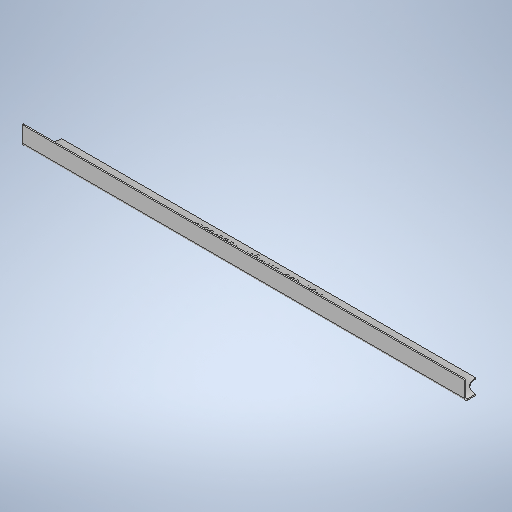
# Autodesk Inventor part: MSC 068 stringer lowerback
Saved by Autodesk Inventor 2025 (Build 290162010, 162A)
## iProperties
Created: 2024-04-28
Part Number: MSC 068 stringer lowerback
Material: Stainless Steel
Document SubType Name: Sheet Metal
Designer: admin
Stock Number: МОО 068 стрингер поясница
Density: 8 g/cm^3
Flat Pattern Width: 70 cm
Flat Pattern Length: 6.6202 cm
Flat Pattern Area: 463.414 cm^2
Sheet Metal Rule: AISI304 2mm Die16
Sheet Metal Width: 700,000 mm
Sheet Metal Length: 66,202 mm
Sheet Metal Area: 46341,393 mm^2
Appearance: Default
Author: admin
Autodesk Inventor part; units mm, degrees
ref_plane "YZ Plane" through (0, 0, 0) normal (1, 0, 0) x (0, 1, 0)
ref_plane "XZ Plane" through (0, 0, 0) normal (0, 1, 0) x (-1, 0, 0)
ref_plane "XY Plane" through (0, 0, 0) normal (0, 0, 1) x (1, 0, 0)
sketch "Sketch1" plane through (0, 0, 0) normal (0, 0, 1) x (1, 0, 0)
  line L0 (-700, 40) -> (0, 40)
  line L1 (0, 40) -> (0, 0)
  line L2 (0, 0) -> (-700, 0)
  line L3 (-700, 0) -> (-700, 40)
  point P0 (-350, 0)
  dimension "d1" = 40
  dimension "d45" = 700
  measures "d1" distance of L0.end L1.end
  measures "d45" distance of L1.end L2.end
extrude "Plate1" add sketch "Sketch1" along normal blind 2
sketch "Sketch2" plane through (0, 2, 0) normal (0, -1, 0) x (1, 0, 0)
  line L0 (-700, 0) -> (0, 0)
  line L1 (0, 0) -> (0, 30)
  line L2 (0, 30) -> (-700, 30)
  line L3 (-700, 30) -> (-700, 0)
  constraints: 6 end point, 1 horizontal, 1 perpendicular, 1 vertical
edge flange "Flange1" height 30 angle 90 thickness 2 bend radius 2.75 thickness toward (0, -1, 0) relief round relief width 2 relief depth 1 edges at (-350, 0, 2) wall of the first edge with corners at (-700, 2, 0) (0, 2, 0) (0, 2, 30) (-700, 2, 30)
bend "Bend1"
corner "Corner1"
sketch "Sketch6" plane through (0, 0, 0) normal (0, 0, -1) x (-1, 0, 0)
  line L0 (0, 40) -> (0, 4.75) projected
  circle A0 centre (0, 40) radius 22.5
  line L1 (0, 40) -> (700, 40) projected
  line L2 (-499, 30) -> (-499, 67.6691) projected
  point P0 (0, 0)
  point P1 (22.5, 40)
  point P2 (0, 17.5)
  dimension "d24" = 45
  constraints: 1 centre point, 1 other
  measures "d24" diameter of A0
extrude "Extrusion2" cut sketch "Sketch6" along normal mid plane 30 contours L1 A0 L0 picked at (14.812, 38.3311)
sketch "Sketch9" plane through (0, 0, 2) normal (0, 0, 1) x (1, 0, 0)
  line L0 (-256.9226, 35) -> (-256.9226, 23) construction
  line L1 (-256.9226, 23) -> (-456.9226, 23) construction
  line L2 (-456.9226, 23) -> (-456.9226, 35) construction
  line L3 (-456.9226, 35) -> (-256.9226, 35) construction
  line L4 (-700, 40) -> (0, 40) projected
  point P0 (0, 0)
  dimension "d40" = 200
  dimension "d41" = 12
  dimension "d43" = 5
  constraints: 2 other
  measures "d40" distance of L0.end L1.end
  measures "d41" distance of L1.end L2.end
  measures "d43" distance between parallel lines of L4 L3
mark "Mark2"
sketch "Sketch10" plane through (-700, 40, 2) normal (0, 0, 1) x (1, 0, 0)
  circle A0 centre (0, 0) radius 22.5
  line L0 (246.5218, -6.4882) -> (246.5218, -9.8215) projected
  line L1 (246.5218, -9.8215) -> (246.5218, -16.4882) projected
  line L2 (246.5218, -9.8215) -> (242.0774, -13.1549) projected
  line L3 (269.8552, -13.1549) -> (269.8552, -6.4882) projected
  line L4 (269.8552, -16.4882) -> (269.8552, -13.1549) projected
  line L5 (267.0774, -13.1549) -> (269.8552, -13.1549) projected
  arc A1 (265.4107, -11.4882) -> (267.0774, -13.1549) centre (267.0774, -11.4882) ccw projected
  line L6 (265.4107, -8.1549) -> (265.4107, -11.4882) projected
  arc A2 (267.0774, -6.4882) -> (265.4107, -8.1549) centre (267.0774, -8.1549) ccw projected
  line L7 (269.8552, -6.4882) -> (267.0774, -6.4882) projected
  line L8 (305.4107, -6.4882) -> (305.9663, -6.4882) projected
  arc A3 (307.6329, -8.1549) -> (305.9663, -6.4882) centre (305.9663, -8.1549) ccw projected
  line L9 (307.6329, -8.1549) -> (307.6329, -16.4882) projected
  circle A4 centre (351.244, -16.2104) radius 0.2778 projected
  line L10 (351.244, -6.4882) -> (351.244, -13.1549) projected
  line L11 (363.744, -6.4882) -> (363.744, -13.1549) projected
  line L12 (364.8552, -13.1549) -> (363.744, -13.1549) projected
  line L13 (363.744, -13.1549) -> (363.744, -16.4882) projected
  line L14 (363.744, -13.1549) -> (361.5218, -13.1549) projected
  line L15 (419.2996, -6.4882) -> (421.5218, -6.4882) projected
  arc A5 (423.744, -8.7104) -> (421.5218, -6.4882) centre (421.5218, -8.7104) ccw projected
  line L16 (423.744, -8.7104) -> (423.744, -14.266) projected
  arc A6 (421.5218, -16.4882) -> (423.744, -14.266) centre (421.5218, -14.266) ccw projected
  line L17 (421.5218, -16.4882) -> (419.2996, -16.4882) projected
  line L18 (442.0774, -6.4882) -> (442.0774, -16.4882) projected
  line L19 (442.0774, -16.4882) -> (438.744, -10.9326) projected
  line L20 (438.744, -10.9326) -> (435.4107, -16.4882) projected
  line L21 (435.4107, -16.4882) -> (435.4107, -6.4882) projected
  arc A7 (432.0774, -7.0437) -> (429.2996, -6.4882) centre (430.0103, -10.157) ccw projected
  arc A8 (429.2996, -6.4882) -> (428.1885, -10.9326) centre (429.3983, -8.874) ccw projected
  line L22 (428.1885, -10.9326) -> (430.9663, -12.5993) projected
  arc A9 (431.5218, -15.9326) -> (430.9663, -12.5993) centre (429.8374, -14.5004) ccw projected
  arc A10 (427.0774, -15.9326) -> (431.5218, -15.9326) centre (429.2996, -11.8029) ccw projected
  arc A11 (402.0774, -15.3771) -> (405.4107, -15.3771) centre (403.744, -14.6897) ccw projected
  arc A12 (402.0774, -7.5993) -> (402.0774, -15.3771) centre (415.5209, -11.4882) ccw projected
  arc A13 (405.4107, -7.5993) -> (402.0774, -7.5993) centre (403.744, -8.308) ccw projected
  arc A14 (405.4107, -15.3771) -> (405.4107, -7.5993) centre (391.9672, -11.4882) ccw projected
  arc A15 (394.8552, -16.4882) -> (398.1885, -10.9326) centre (392.4255, -11.2526) ccw projected
  line L23 (398.1885, -10.9326) -> (398.1885, -8.7104) projected
  arc A16 (398.1885, -8.7104) -> (393.744, -8.7104) centre (395.9663, -8.7104) ccw projected
  line L24 (393.744, -8.7104) -> (393.744, -9.8215) projected
  arc A17 (393.744, -9.8215) -> (395.9663, -12.0437) centre (395.9663, -9.8215) ccw projected
  line L25 (395.9663, -12.0437) -> (397.6329, -12.0437) projected
  line L26 (385.9663, -8.7104) -> (385.9663, -9.8215) projected
  arc A18 (390.4107, -8.7104) -> (385.9663, -8.7104) centre (388.1885, -8.7104) ccw projected
  line L27 (390.4107, -9.8215) -> (390.4107, -8.7104) projected
  arc A19 (388.1885, -12.0437) -> (390.4107, -9.8215) centre (388.1885, -9.8215) ccw projected
  line L28 (388.744, -12.0437) -> (388.1885, -12.0437) projected
  arc A20 (390.4107, -13.7104) -> (388.744, -12.0437) centre (388.744, -13.7104) ccw projected
  line L29 (390.4107, -14.8215) -> (390.4107, -13.7104) projected
  arc A21 (388.744, -16.4882) -> (390.4107, -14.8215) centre (388.744, -14.8215) ccw projected
  line L30 (387.6329, -16.4882) -> (388.744, -16.4882) projected
  arc A22 (385.9663, -14.8215) -> (387.6329, -16.4882) centre (387.6329, -14.8215) ccw projected
  line L31 (385.9663, -13.7104) -> (385.9663, -14.8215) projected
  arc A23 (387.6329, -12.0437) -> (385.9663, -13.7104) centre (387.6329, -13.7104) ccw projected
  line L32 (388.1885, -12.0437) -> (387.6329, -12.0437) projected
  arc A24 (385.9663, -9.8215) -> (388.1885, -12.0437) centre (388.1885, -9.8215) ccw projected
  arc A25 (372.6329, -7.5993) -> (370.9663, -6.4882) centre (370.9544, -8.3116) ccw projected
  line L33 (370.9663, -6.4882) -> (369.8552, -6.4882) projected
  arc A26 (369.8552, -6.4882) -> (368.1885, -7.5993) centre (369.8671, -8.3116) ccw projected
  line L34 (368.1885, -7.5993) -> (368.1885, -8.1549) projected
  arc A27 (368.1885, -8.1549) -> (369.2996, -9.266) centre (370.044, -7.4104) ccw projected
  line L35 (369.2996, -9.266) -> (371.5218, -10.3771) projected
  arc A28 (372.6329, -11.4882) -> (371.5218, -10.3771) centre (370.7774, -12.2326) ccw projected
  line L36 (372.6329, -11.4882) -> (372.6329, -12.0437) projected
  arc A29 (370.9663, -13.1549) -> (372.6329, -12.0437) centre (370.9544, -11.3314) ccw projected
  line L37 (370.9663, -13.1549) -> (369.8552, -13.1549) projected
  arc A30 (368.1885, -12.0437) -> (369.8552, -13.1549) centre (369.8671, -11.3314) ccw projected
  line L38 (358.1885, -6.4882) -> (358.1885, -13.1549) projected
  line L39 (358.1885, -13.1549) -> (355.9663, -13.1549) projected
  arc A31 (354.8552, -12.0437) -> (355.9663, -13.1549) centre (355.9663, -12.0437) ccw projected
  line L40 (347.6329, -6.4882) -> (347.6329, -13.1549) projected
  line L41 (347.6329, -13.1549) -> (344.8552, -13.1549) projected
  arc A32 (343.1885, -11.4882) -> (344.8552, -13.1549) centre (344.8552, -11.4882) ccw projected
  line L42 (343.1885, -11.4882) -> (343.1885, -6.4882) projected
  line L43 (338.1885, -13.1549) -> (335.4107, -13.1549) projected
  line L44 (335.4107, -13.1549) -> (335.4107, -6.4882) projected
  line L45 (335.4107, -6.4882) -> (335.4107, -4.8215) projected
  arc A33 (337.0774, -3.1549) -> (335.4107, -4.8215) centre (337.0774, -4.8215) ccw projected
  line L46 (337.0774, -3.1549) -> (339.8552, -3.1549) projected
  line L47 (335.4107, -6.4882) -> (338.1885, -6.4882) projected
  arc A34 (339.8552, -8.1549) -> (338.1885, -6.4882) centre (338.1885, -8.1549) ccw projected
  line L48 (339.8552, -8.1549) -> (339.8552, -11.4882) projected
  arc A35 (338.1885, -13.1549) -> (339.8552, -11.4882) centre (338.1885, -11.4882) ccw projected
  line L49 (332.0774, -10.9326) -> (332.0774, -9.8215) projected
  arc A36 (327.6329, -10.9326) -> (332.0774, -10.9326) centre (329.8552, -10.9326) ccw projected
  line L50 (327.6329, -9.8215) -> (327.6329, -10.9326) projected
  line L51 (332.0774, -9.8215) -> (327.6329, -9.8215) projected
  line L52 (332.0774, -9.8215) -> (332.0774, -8.1549) projected
  arc A37 (332.0774, -8.1549) -> (330.4107, -6.4882) centre (330.4107, -8.1549) ccw projected
  line L53 (330.4107, -6.4882) -> (327.6329, -6.4882) projected
  line L54 (324.2996, -6.4882) -> (324.2996, -13.1549) projected
  line L55 (324.2996, -13.1549) -> (322.0774, -13.1549) projected
  arc A38 (320.9663, -12.0437) -> (322.0774, -13.1549) centre (322.0774, -12.0437) ccw projected
  arc A39 (297.6329, -10.9326) -> (302.0774, -10.9326) centre (299.8552, -10.9326) ccw projected
  line L56 (297.6329, -8.7104) -> (297.6329, -10.9326) projected
  arc A40 (302.0774, -8.7104) -> (297.6329, -8.7104) centre (299.8552, -8.7104) ccw projected
  line L57 (302.0774, -10.9326) -> (302.0774, -8.7104) projected
  line L58 (294.2996, -13.1549) -> (292.6329, -6.4882) projected
  line L59 (292.6329, -6.4882) -> (290.9663, -10.9326) projected
  line L60 (290.9663, -10.9326) -> (289.2996, -6.4882) projected
  line L61 (289.2996, -6.4882) -> (287.6329, -13.1549) projected
  line L62 (284.2996, -10.9326) -> (284.2996, -9.8215) projected
  arc A41 (279.8552, -10.9326) -> (284.2996, -10.9326) centre (282.0774, -10.9326) ccw projected
  line L63 (279.8552, -9.8215) -> (279.8552, -10.9326) projected
  line L64 (284.2996, -9.8215) -> (279.8552, -9.8215) projected
  line L65 (284.2996, -9.8215) -> (284.2996, -8.1549) projected
  arc A42 (284.2996, -8.1549) -> (282.6329, -6.4882) centre (282.6329, -8.1549) ccw projected
  line L66 (282.6329, -6.4882) -> (279.8552, -6.4882) projected
  line L67 (276.5218, -6.4882) -> (276.5218, -13.1549) projected
  line L68 (276.5218, -13.1549) -> (274.2996, -13.1549) projected
  arc A43 (273.1885, -12.0437) -> (274.2996, -13.1549) centre (274.2996, -12.0437) ccw projected
  line L69 (259.8552, -13.1549) -> (257.6329, -13.1549) projected
  line L70 (257.6329, -13.1549) -> (257.6329, -8.1549) projected
  line L71 (257.6329, -8.1549) -> (257.6329, -7.5993) projected
  arc A44 (257.6329, -7.5993) -> (256.5218, -6.4882) centre (256.5218, -7.5993) ccw projected
  arc A45 (259.2996, -6.4882) -> (257.6329, -8.1549) centre (259.2996, -8.1549) ccw projected
  line L72 (259.2996, -6.4882) -> (260.4107, -6.4882) projected
  arc A46 (262.0774, -8.1549) -> (260.4107, -6.4882) centre (260.4107, -8.1549) ccw projected
  line L73 (262.0774, -8.1549) -> (262.0774, -10.9326) projected
  arc A47 (259.8552, -13.1549) -> (262.0774, -10.9326) centre (259.8552, -10.9326) ccw projected
  line L74 (249.8552, -6.4882) -> (251.5218, -6.4882) projected
  arc A48 (253.1885, -8.1549) -> (251.5218, -6.4882) centre (251.5218, -8.1549) ccw projected
  line L75 (253.1885, -8.1549) -> (253.1885, -11.4882) projected
  arc A49 (251.5218, -13.1549) -> (253.1885, -11.4882) centre (251.5218, -11.4882) ccw projected
  line L76 (251.5218, -13.1549) -> (249.8552, -13.1549) projected
  line L77 (244.8552, -10.9326) -> (242.0774, -6.4882) projected
  arc A50 (677.5, 0) -> (700, -22.5) centre (700, 0) ccw projected
  line L78 (0, 0) -> (677.5, 0) projected
  line L79 (0, -35.25) -> (0, 0) projected
  line L80 (0, -35.25) -> (700, -35.25) projected
  line L81 (700, -22.5) -> (700, -35.25) projected
  point P0 (700, -40)
  point P1 (0, -22.5)
  point P2 (22.5, 0)
  dimension "d46" = 45
  constraints: 1 centre point, 1 coincident
  measures "d46" diameter of A0
extrude "Extrusion4" cut sketch "Sketch10" against normal through all contours A0 L79 L78 picked at (14.812, -1.6689)
equation "\"d43\" = d42"
equation "\"d2\" = Thickness"
equation "\"d3\" = BendReliefWidth"
equation "\"d4\" = BendReliefDepth"
equation "\"d5\" = MinimumRemnant"
equation "\"d6\" = TransitionRadius"
equation "\"d9\" = BendRadius"
equation "\"d10\" = CornerReliefSize"
equation "\"d11\" = GapSize"
equation "\"d12\" = JacobiRadiusSize"
equation "\"BendReliefWidth\" = Thickness"
equation "\"BendReliefDepth\" = 0.5 * Thickness"
equation "\"CornerReliefSize\" = 4 * Thickness"
equation "\"MinimumRemnant\" = 2 * Thickness"
equation "\"TransitionRadius\" = BendRadius"
equation "\"JacobiRadiusSize\" = BendRadius"
equation "\"GapSize\" = Thickness"
equation "\"qqqqqq\" = 67.35706"
equation "\"d42\" = 5"
equation "\"Thickness\" = 2"
equation "\"BendRadius\" = 2.75"
body "Solid1"
